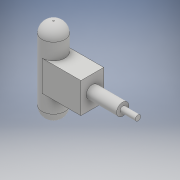
# Autodesk Inventor part: Mic
Saved by Autodesk Inventor 2017 (Build 210142000, 142)
## iProperties
Created: 2017-06-02
Part Number: Mic
Material: Generic
Document SubType Name: Modeling
Designer: crush
Density: 1 g/cm^3
Appearance: Default
Author: crush
Autodesk Inventor part; units mm, degrees
ref_plane "YZ Plane" through (0, 0, 0) normal (1, 0, 0) x (0, 1, 0)
ref_plane "XZ Plane" through (0, 0, 0) normal (0, 1, 0) x (-1, 0, 0)
ref_plane "XY Plane" through (0, 0, 0) normal (0, 0, 1) x (1, 0, 0)
sketch "Sketch1" plane through (0, 0, 0) normal (0, 0, 1) x (1, 0, 0)
  circle A0 centre (0, 0) radius 7.5
  dimension "d0" = 15
  constraints: 1 centre point, 1 coincident
  measures "d0" diameter of A0
extrude "Extrusion1" add sketch "Sketch1" along normal blind 55
fillet "Fillet1" radius 7 1 edges at (-7.5, 0, 55)
fillet "Fillet2" radius 7 1 edges at (-7.5, 0, 0)
sketch "Sketch2" plane through (0, 0, 0) normal (1, 0, 0) x (0, 1, 0)
  line L0 (-7.5, 7) -> (-7.5, 48) projected
  line L1 (-7.5, 37.3739) -> (7.5, 37.3739)
  line L2 (7.5, 37.3739) -> (7.5, 17.3739)
  line L3 (7.5, 17.3739) -> (-7.5, 17.3739)
  line L4 (-7.5, 17.3739) -> (-7.5, 37.3739)
  point P0 (0, 0)
  dimension "d5" = 15
  dimension "d6" = 20
  constraints: 8 end point, 2 parallel, 1 horizontal, 1 perpendicular, 1 point on line
  measures "d5" distance of L2.end L3.end
  measures "d6" distance of L1.end L2.end
extrude "Extrusion2" add sketch "Sketch2" along normal blind 25.5
sketch "Sketch3" plane through (25.5, 0, 0) normal (1, 0, 0) x (0, 0, -1)
  line L0 (-37.3739, 7.5) -> (-37.3739, -7.5) projected
  line L1 (-37.3739, 0) -> (-27.3739, 0)
  circle A0 centre (-27.3739, 0) radius 1.75
  point P0 (0, 0)
  dimension "d9" = 10
  dimension "d10" = 3.5
  constraints: 2 end point, 1 centre point, 1 coincident, 1 horizontal, 1 midpoint
  measures "d9" distance of L1.start L1.end
  measures "d10" diameter of A0
extrude "Extrusion3" add sketch "Sketch3" along normal blind 30
sketch "Sketch4" plane through (25.5, 0, 0) normal (1, 0, 0) x (0, 0, -1)
  circle A0 centre (-27.3739, 0) radius 1.75 projected
  circle A1 centre (-27.3739, 0) radius 4
  point P0 (0, 0)
  dimension "d13" = 8
  constraints: 1 centre point, 1 coincident
  measures "d13" diameter of A1
extrude "Extrusion4" add sketch "Sketch4" along normal blind 20
body "Solid1"
